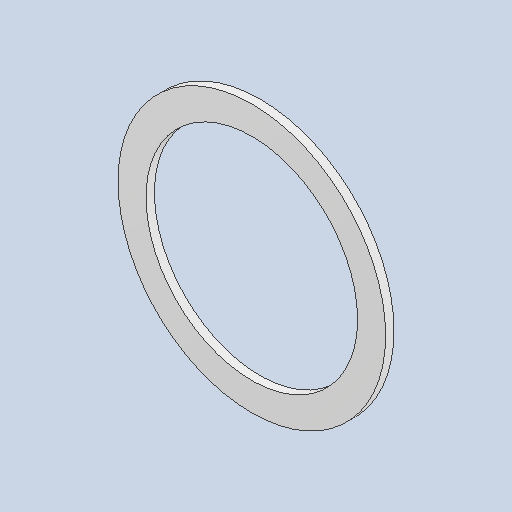
# Autodesk Inventor part: TT-2532-10
Saved by Autodesk Inventor 2022.4 (Build 264492000, 492)
## iProperties
Created: 2021-09-28
Part Number: TT-2532-10
Material: PET プラスチック
Document SubType Name: Modeling
Designer: Masato
Density: 1.541 g/cm^3
Appearance: 滑らか - 白
Description: 既製品
Mass: 0.464646 g
Surface Area: 7.83058 cm^2
Volume: 0.301522 cm^3
Author: Masato Kubotera
Comments: https://www.hirosugi-net.co.jp/shop/g/g32088/
Autodesk Inventor part; units mm, degrees
ref_plane "YZ Plane" through (0, 0, 0) normal (1, 0, 0) x (0, 1, 0)
ref_plane "XZ Plane" through (0, 0, 0) normal (0, 1, 0) x (-1, 0, 0)
ref_plane "XY Plane" through (0, 0, 0) normal (0, 0, 1) x (1, 0, 0)
sketch "スケッチ1" plane through (0, 0, 0) normal (0, 0, 1) x (1, 0, 0)
  circle A0 centre (0, 0) radius 12.65
  circle A1 centre (0, 0) radius 16
  dimension "d0" = 25.3
  dimension "d1" = 32
  constraints: 2 centre point, 2 coincident
  measures "d0" diameter of A0
  measures "d1" diameter of A1
extrude "押し出し1" add sketch "スケッチ1" along normal blind 1
